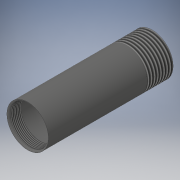
# Autodesk Inventor part: badan lampu
Saved by Autodesk Inventor 2019.5 (Build 235369000, 369)
## iProperties
Created: 2022-10-10
Part Number: badan lampu
Material: Aluminum 6061-AHC
Document SubType Name: Modeling
Designer: ASUS
Density: 2.7 g/cm^3
Appearance: Aluminum - Dark
Author: ASUS
Autodesk Inventor part; units mm, degrees
ref_plane "YZ Plane" through (0, 0, 0) normal (1, 0, 0) x (0, 1, 0)
ref_plane "XZ Plane" through (0, 0, 0) normal (0, 1, 0) x (-1, 0, 0)
ref_plane "XY Plane" through (0, 0, 0) normal (0, 0, 1) x (1, 0, 0)
sketch "Sketch1" plane through (0, 0, 0) normal (0, 0, 1) x (1, 0, 0)
  circle A0 centre (0, 0) radius 20
  dimension "d0" = 40
  constraints: 1 centre point, 1 coincident
  measures "d0" diameter of A0
extrude "Extrusion1" add sketch "Sketch1" along normal blind 120
sketch "Sketch2" plane through (0, 0, 0) normal (0, 0, -1) x (-1, 0, 0)
  point P0 (0, 0)
  point P1 (0, 0)
  constraints: 1 coincident
hole "Hole1" at (0, 0, 0) at (0, 0, 0) direction (0, 0, 1) diameter 35 depth 86.25
shell "Shell1" thickness 1.5 removed faces 1 at (-2.364, 6.2334, 120)
sketch "Sketch3" plane through (0, 0, 87.75) normal (0, 0, 1) x (1, 0, 0)
  point P0 (0, 0)
  point P1 (-0.8402, 0.3734)
hole "Hole2" at (-0.8402, 0.3734, 87.75) direction (0, 0, -1) diameter 10 depth 86.25
fillet "Fillet1" radius 2 1 edges at (-18.5, 0, 120)
thread "Thread1" size "M40x3" class "6g" standard "ANSI Metric M Profile" length 25
thread "Thread2" size "M38x1.5" class "6H" standard "ANSI Metric M Profile" length 10
body "Solid1"
